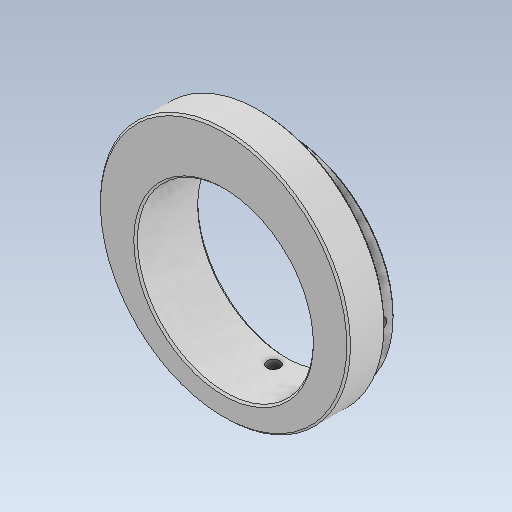
# Autodesk Inventor part: Peça23
Saved by Autodesk Inventor 2021 (Build 250183000, 183)
## iProperties
Category: 41
Created: 2021-07-19
Part Number: Peça23
Material: Genérico
Document SubType Name: Modeling
Designer: Giovanni
Density: 1 g/cm^3
Appearance: Padrão
User Status: 1:3
Author: Giovanni
Keywords: 29
Autodesk Inventor part; units mm, degrees
ref_plane "YZ Plane" through (0, 0, 0) normal (1, 0, 0) x (0, 1, 0)
ref_plane "XZ Plane" through (0, 0, 0) normal (0, 1, 0) x (-1, 0, 0)
ref_plane "XY Plane" through (0, 0, 0) normal (0, 0, 1) x (1, 0, 0)
sketch "Esboço1" plane through (0, 0, 0) normal (0, 0, 1) x (1, 0, 0)
  circle A0 centre (0, 0) radius 47.5
  circle A1 centre (0, 0) radius 57.5
  dimension "d0" = 95
  dimension "d1" = 115
  constraints: 2 centre point, 2 coincident
  measures "d0" diameter of A0
  measures "d1" diameter of A1
extrude "Extrusão1" add sketch "Esboço1" against normal blind 15
sketch "Esboço2" plane through (0, 0, 0) normal (0, 0, 1) x (1, 0, 0)
  circle A0 centre (0, 8) radius 67.5
  circle A1 centre (0, 0) radius 47.5 projected
  dimension "d4" = 135
  dimension "d5" = 8
  constraints: 1 centre point
  measures "d4" diameter of A0
  measures "d5" distance of point (0, 0) A0.centre
extrude "Extrusão2" add sketch "Esboço2" along normal blind 20
sketch "Esboço3" plane through (0, 0, 0) normal (0, 1, 0) x (-1, 0, 0)
  line L0 (47.5, -15) -> (-47.5, -15) projected
  point P0 (0, 0)
  point P1 (0, -7)
  point P2 (0, -15)
  dimension "d8" = 8
  constraints: 1 midpoint, 1 vertical alignment
  measures "d8" distance from line of L0 point (0, -7)
hole "Furo1" at (0, 0, -7) direction (0, -1, 0) diameter 6.917 end through all thread size "M8x1" class "6H" standard "ANSI Metric M Profile"
chamfer "Chanfro1" distance 0.5 angle 45 1 edges at (-0.0571, -57.5, -10.458)
pattern_circular "Padrão circular1" count 2 over 90 about axis through (0, 0, -10) along (0, 0, 1) of "Furo1"
chamfer "Chanfro2" distance 1.5 angle 45 1 edges at (-47.5, 0, -15)
chamfer "Chanfro3" distance 1 angle 45 5 edges at (-57.5, 0, -15) (-57.5, 0, 0) (-67.5, 8, 0) (-67.5, 8, 20) (-47.5, 0, 20)
